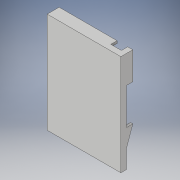
# Autodesk Inventor part: Enclosure
Saved by Autodesk Inventor 2017.3 (Build 213256000, 256)
## iProperties
Created: 2018-08-13
Part Number: Enclosure
Material: Generic
Document SubType Name: Modeling
Designer: Michael
Density: 1 g/cm^3
Appearance: Default
Author: Michael
Autodesk Inventor part; units mm, degrees
ref_plane "YZ Plane" through (0, 0, 0) normal (1, 0, 0) x (0, 1, 0)
ref_plane "XZ Plane" through (0, 0, 0) normal (0, 1, 0) x (-1, 0, 0)
ref_plane "XY Plane" through (0, 0, 0) normal (0, 0, 1) x (1, 0, 0)
sketch "Sketch1" plane through (0, 0, 0) normal (0, 1, 0) x (-1, 0, 0)
  line L0 (58.83, 0) -> (0, 0)
  line L1 (0, 0) -> (0, -81.82)
  line L2 (0, -81.82) -> (58.83, -81.82)
  line L3 (58.83, -81.82) -> (58.83, 0)
  point P0 (0, 0)
  dimension "d0" = 58.83
  dimension "d1" = 81.82
  constraints: 8 end point, 2 parallel, 1 horizontal, 1 perpendicular
  measures "d0" distance of L2.end L1.end
  measures "d1" distance of L1.end L0.end
extrude "Extrusion1" add sketch "Sketch1" along normal blind 1
sketch "Sketch2" plane through (0, 1, 0) normal (0, 1, 0) x (1, 0, 0)
  line L0 (-56.83, 0) -> (-58.83, 2)
  line L1 (-56.83, 81.82) -> (-58.83, 79.82)
  line L2 (0, 79.82) -> (-2, 81.82)
  line L3 (-2, 0) -> (0, 2)
  line L4 (-58.83, 0) -> (0, 0) projected
  line L5 (-58.83, 0) -> (-58.83, 2)
  line L6 (-58.83, 81.82) -> (-58.83, 0) projected
  line L7 (-58.83, 0) -> (-56.83, 0)
  line L8 (-58.83, 81.82) -> (-58.83, 79.82)
  line L9 (-58.83, 2) -> (-58.83, 0)
  line L10 (-58.83, 0) -> (-56.83, 0)
  line L11 (-2, 0) -> (0, 0)
  line L12 (0, 0) -> (0, 2)
  line L13 (0, 79.82) -> (0, 81.82)
  line L14 (0, 81.82) -> (-2, 81.82)
  line L15 (-56.83, 81.82) -> (-58.83, 81.82)
  dimension "d4" = 2
  dimension "d5" = 2
  dimension "d6" = 2
  dimension "d7" = 2
  dimension "d8" = 2
  dimension "d9" = 2
  dimension "d10" = 2
  dimension "d11" = 2
  constraints: 28 end point, 2 collinear
  measures "d4" distance of L0.start L4.start
  measures "d5" distance of L0.end L4.start
  measures "d6" distance of L1.start L6.start
  measures "d7" distance of L1.end L6.start
  measures "d8" distance of L2.start point (0, 81.82)
  measures "d9" distance of L2.end point (0, 81.82)
  measures "d10" distance of L3.start point (0, 0)
  measures "d11" distance of L3.end point (0, 0)
extrude "Extrusion2" add sketch "Sketch2" along normal blind 2.2
sketch "Sketch3" plane through (0, 0, 0) normal (0, -1, 0) x (1, 0, 0)
  line L0 (-58.83, 0) -> (0, 0) projected
  line L1 (-58.83, -81.82) -> (-58.83, 0) projected
  line L2 (0, -81.82) -> (-58.83, -81.82) projected
  line L3 (0, 0) -> (0, -81.82) projected
  line L4 (2, 2) -> (-60.83, 2)
  line L5 (-60.83, 2) -> (-60.83, -83.82)
  line L6 (-60.83, -83.82) -> (2, -83.82)
  line L7 (2, -83.82) -> (2, 2)
  point P0 (0, 0)
  dimension "d14" = 2
  constraints: 8 end point, 3 other
  measures "d14" distance between parallel lines of L0 L4
extrude "Extrusion3" add sketch "Sketch3" against normal blind 10.2
sketch "Sketch4" plane through (0, 10.2, 0) normal (0, 1, 0) x (1, 0, 0)
  line L0 (-58.83, 0) -> (-58.83, 81.82) projected
  line L1 (-58.83, 81.82) -> (0, 81.82) projected
  line L2 (0, 81.82) -> (0, 0) projected
  line L3 (0, 0) -> (-58.83, 0) projected
  line L4 (-60.83, -2) -> (2, -2) projected
  line L5 (2, -2) -> (2, 83.82) projected
  line L6 (2, 83.82) -> (-60.83, 83.82) projected
  line L7 (-60.83, 83.82) -> (-60.83, -2) projected
  line L8 (0, 0) -> (-2.3, 0)
  line L9 (-56.83, 0) -> (-2, 0) projected
  line L10 (2, -2) -> (-60.83, -2) projected
  line L11 (-2.3, 0) -> (-11.35, 0)
  line L12 (-11.35, 0) -> (-11.35, -2)
  line L13 (-11.35, -2) -> (-2.3, -2)
  line L14 (-2.3, -2) -> (-2.3, 0)
  point P0 (0, 0)
  dimension "d17" = 2.3
  dimension "d18" = 9.05
  constraints: 10 end point, 2 parallel, 2 point on line, 1 horizontal, 1 perpendicular
  measures "d17" distance of L2.end L8.end
  measures "d18" distance of L13.end L12.end
extrude "Extrusion4" cut sketch "Sketch4" against normal blind 7 contours L3 L14 L4 L12
sketch "Sketch5" plane through (0, 10.2, 0) normal (0, 1, 0) x (1, 0, 0)
  line L0 (0, 0) -> (0, 21.65)
  line L1 (0, 81.82) -> (0, 0) projected
  line L2 (2, -2) -> (2, 83.82) projected
  line L3 (0, 21.65) -> (2, 21.65)
  line L4 (2, 21.65) -> (2, 52.75)
  line L5 (2, 52.75) -> (0, 52.75)
  line L6 (0, 52.75) -> (0, 21.65)
  dimension "d21" = 21.65
  dimension "d22" = 31.1
  constraints: 10 end point, 2 parallel, 2 point on line, 1 horizontal, 1 perpendicular
  measures "d21" distance of L0.start L0.end
  measures "d22" distance of L4.end L3.end
extrude "Extrusion5" cut sketch "Sketch5" against normal blind 7
sketch "Sketch7" plane through (0, 3.2, -81.82) normal (-1, 0, 0) x (0, 0, 1)
  line L0 (60.17, 7) -> (60.17, 0) projected
  line L1 (60.17, 0) -> (29.07, 0) projected
  line L2 (29.07, 0) -> (29.07, 7) projected
  line L3 (0, 7) -> (29.07, 7) projected
  line L4 (2, -2.2) -> (2, 0) projected
  line L5 (79.82, -2.2) -> (2, -2.2) projected
  line L6 (79.82, -2.2) -> (79.82, 0) projected
  line L7 (81.82, 0) -> (79.82, 0) projected
  line L8 (81.82, 0) -> (81.82, 7) projected
  line L9 (60.17, 7) -> (81.82, 7) projected
  line L10 (0, 0) -> (0, 1.6)
  line L11 (0, 0) -> (0, 7) projected
  line L12 (0, 1.6) -> (13.65, 1.6)
  line L13 (29.07, 7) -> (29.07, 0) projected
  line L14 (13.65, 1.6) -> (29.07, 7)
  line L15 (29.07, 7) -> (-2, 7) projected
  line L16 (29.07, 7) -> (-2, 7)
  line L17 (-2, 7) -> (-2, 1.6)
  line L18 (-2, 1.6) -> (0, 1.6)
  point P0 (81.82, -3.2)
  dimension "d25" = 1.6
  dimension "d26" = 13.65
  dimension "d27" = 90
  constraints: 13 end point, 2 point on line, 1 horizontal, 1 parallel
  measures "d25" distance of L10.start L10.end
  measures "d26" distance of L10.end L12.end
  measures "d27" angle of L10 L12
extrude "Extrusion6" cut sketch "Sketch7" against normal blind 7 and the other way blind 61 contours L3 L14 L12 L11
sketch "Sketch8" plane through (-60.83, 0, -83.82) normal (-1, 0, 0) x (0, 0, 1)
  line L0 (2, 4.8) -> (15.65, 4.8) projected
  line L1 (15.65, 4.8) -> (31.07, 10.2) projected
  line L2 (31.07, 10.2) -> (85.82, 10.2) projected
  line L3 (85.82, 10.2) -> (85.82, 0) projected
  line L4 (85.82, 0) -> (0, 0) projected
  line L5 (0, 0) -> (0, 10.2) projected
  line L6 (0, 10.2) -> (2, 10.2) projected
  line L7 (2, 10.2) -> (2, 4.8) projected
  line L8 (2, 4.8) -> (2, 10.2) projected
  line L9 (0, 10.2) -> (2, 10.2) projected
  line L10 (0, 0) -> (0, 10.2) projected
  line L11 (85.82, 0) -> (0, 0) projected
  line L12 (85.82, 0) -> (85.82, 10.2) projected
  line L13 (31.07, 10.2) -> (85.82, 10.2) projected
  line L14 (31.07, 10.2) -> (15.65, 4.8) projected
  line L15 (15.65, 4.8) -> (2, 4.8) projected
  line L16 (0, 10.2) -> (2, 10.2) projected
  line L17 (0, 10.2) -> (2, 10.2)
  line L18 (2, 10.2) -> (2, 4.8)
  line L19 (2, 4.8) -> (0, 4.8)
  line L20 (0, 4.8) -> (0, 10.2)
  point P0 (83.82, 0)
  constraints: 8 end point, 2 parallel, 1 horizontal, 1 perpendicular
extrude "Extrusion7" cut sketch "Sketch8" against normal blind 63 contours L19 L5 L6 L7
sketch "Sketch9" plane through (0, 3.2, 0) normal (0, 1, 0) x (1, 0, 0)
  line L0 (-11.35, 0) -> (-2.3, 0) projected
  line L1 (-11.35, -2) -> (-11.35, 0) projected
  line L2 (-2.3, -2) -> (-11.35, -2) projected
  line L3 (-2.3, 0) -> (-2.3, -2) projected
  line L4 (2, 21.65) -> (0, 21.65) projected
  line L5 (2, 52.75) -> (2, 21.65) projected
  line L6 (0, 52.75) -> (2, 52.75) projected
  line L7 (0, 21.65) -> (0, 52.75) projected
  point P0 (0, 0)
extrude "Extrusion8" add sketch "Sketch9" along normal blind 1.6
equation "\"d5\" = d4"
equation "\"d6\" = d4"
equation "\"d7\" = d6"
equation "\"d8\" = d4"
equation "\"d9\" = d8"
equation "\"d10\" = d4"
equation "\"d11\" = d10"
body "Solid1"
